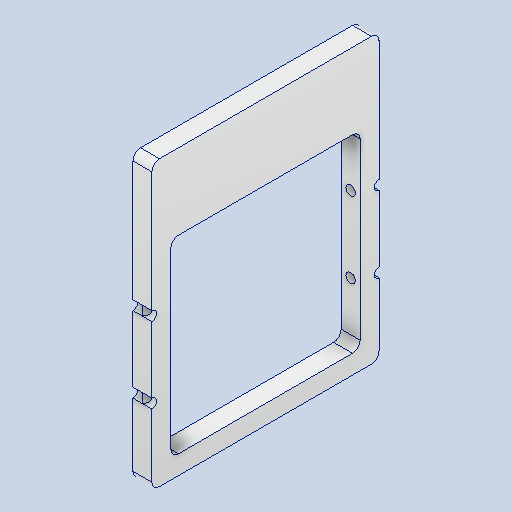
# Autodesk Inventor part: base_weel-v3-Plate-12
Saved by Autodesk Inventor 2025.2 (Build 292293000, 293)
## iProperties
Created: 2025-04-05
Part Number: base_weel-v3-Plate-12
Material: アルミニウム 6061
Document SubType Name: Modeling
Designer: haruy
Density: 2.7 g/cm^3
Appearance: アルミニウム - フラット
Author: haruy
Autodesk Inventor part; units mm, degrees
ref_plane "YZ Plane" through (0, 0, 0) normal (1, 0, 0) x (0, 1, 0)
ref_plane "XZ Plane" through (0, 0, 0) normal (0, 1, 0) x (-1, 0, 0)
ref_plane "XY Plane" through (0, 0, 0) normal (0, 0, 1) x (1, 0, 0)
derived "base_weel-v3-Plate-8.ipt"
sketch "スケッチ9" plane through (0, -300, -190) normal (1, 0, 0) x (0, 0, -1)
  line L0 (-215, 0) -> (-165, 0) projected
  line L1 (-165, 0) -> (-165, -50) projected
  line L2 (-165, -50) -> (-215, -50) projected
  line L3 (-215, -50) -> (-215, 0) projected
  circle A0 centre (-190, -25) radius 22 projected
  line L4 (-212, -25) -> (-168, -25) projected
  line L5 (-380, 0) -> (0, 0) projected
  line L6 (-268.5, 20) -> (-268.5, 241.5) projected
  line L7 (-220, 20) -> (-160, 20) projected
  line L8 (-160, 20) -> (-160, -55) projected
  line L9 (-160, -55) -> (-220, -55) projected
  line L10 (-220, -55) -> (-220, 20) projected
  circle A1 centre (-170, -5) radius 1.5 projected
  line L11 (0, 20) -> (-380, 20) projected
  circle A2 centre (-210, 10) radius 1.25 projected
  circle A3 centre (-190, 10) radius 1.25 projected
  circle A4 centre (-210, -45) radius 1.5 projected
  circle A5 centre (-190, 300) radius 360 projected
  circle A6 centre (-210, -45) radius 1.6 projected
  circle A7 centre (-170, 10) radius 1.25 projected
  circle A8 centre (-190, -25) radius 10 projected
  line L12 (-215, -50) -> (-190, -25) projected
  line L13 (-218.5355, -46.4645) -> (-193.5355, -21.4645) projected
  line L14 (-211.4645, -53.5355) -> (-186.4645, -28.5355) projected
  line L15 (-190, -25) -> (-190, -50) projected
  line L16 (-168.5355, -53.5355) -> (-193.5355, -28.5355) projected
  line L17 (-161.4645, -46.4645) -> (-186.4645, -21.4645) projected
  line L18 (-218.5355, -3.5355) -> (-193.5355, -28.5355) projected
  line L19 (-211.4645, 3.5355) -> (-186.4645, -21.4645) projected
  line L20 (-168.5355, 3.5355) -> (-193.5355, -21.4645) projected
  line L21 (-161.4645, -3.5355) -> (-186.4645, -28.5355) projected
extrude "押し出し1" add sketch "スケッチ9" against normal blind 5 contours L5 L10 L7 L8 L0 | L3 L2 L1 L5 L8 L9 L10 | A2 | A3 | A7
fillet "フィレット1" radius 2 8 edges at (-2.5, -300, -25) (-2.5, -350, -25) (-2.5, -350, 25) (-2.5, -300, 25) (-2.5, -355, 30) (-2.5, -355, -30) (-2.5, -280, -30) (-2.5, -280, 30)
sketch "スケッチ2" plane through (0, -353, 30) normal (0, 0, 1) x (1, 0, 0)
  circle A0 centre (-2.5, 18) radius 1.25
  circle A1 centre (-2.5, 28) radius 1.25
  circle A2 centre (-2.5, 38) radius 1.25
  line L0 (-5, -2) -> (0, -2) projected
  line L1 (-5, 0) -> (-5, 71) projected
  point P0 (0, 353)
  dimension "d4" = 2.5
  dimension "d5" = 2.5
  dimension "d6" = 2.5
  dimension "d7" = 20
  dimension "d8" = 10
  dimension "d9" = 10
  dimension "d10" = 2.5
  dimension "d11" = 2.5
  dimension "d12" = 2.5
  constraints: 3 centre point
  measures "d4" diameter of A0
  measures "d5" diameter of A1
  measures "d6" diameter of A2
  measures "d7" distance from line of A0.centre L0
  measures "d8" distance of A0.centre A1.centre
  measures "d9" distance of A1.centre A2.centre
  measures "d10" distance from line of A2.centre L1
  measures "d11" distance from line of A1.centre L1
  measures "d12" distance from line of A0.centre L1
hole "穴1" at (-2.5, -315, 30) at (-2.5, -335, 30) direction (0, 0, -1) diameter 2.5 end through all
sketch "スケッチ3" plane through (0, -353, 30) normal (1, 0, 0) x (0, 0, -1)
  line L0 (0, 0) -> (0, 71) projected
  circle A0 centre (0, 38) radius 1.25
  circle A1 centre (0, 18) radius 1.25
  line L1 (2, -2) -> (58, -2) projected
  line L2 (5, 5) -> (5, 51) projected
  line L3 (2, 73) -> (58, 73) projected
  line L4 (30, 73) -> (30, -2)
  circle A2 centre (60, 38) radius 1.25
  circle A3 centre (60, 18) radius 1.25
  point P0 (30, 353)
  dimension "d20" = 2.5
  dimension "d21" = 2.5
  dimension "d22" = 20
  dimension "d23" = 20
  dimension "d24" = 5
  constraints: 4 centre point, 2 end point, 2 midpoint, 2 symmetric about line, 1 point on line, 2 other
  measures "d20" diameter of A0
  measures "d21" diameter of A1
  measures "d22" distance from line of A1.centre L1
  measures "d23" distance of A0.centre A1.centre
  measures "d24" distance from line of L2 A1.centre
extrude "押し出し2" cut sketch "スケッチ3" against normal blind 10
equation "\"d9\" = d8"
equation "\"d12\" = d10"
equation "\"d23\" = d22"
